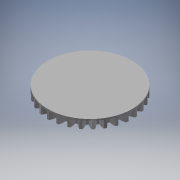
# Autodesk Inventor part: Stirnzahnrad1
Saved by Autodesk Inventor 2018 (Build 220112000, 112)
## iProperties
Created: 2018-01-27
Part Number: Stirnzahnrad1
Material: Steel
Document SubType Name: Modeling
Designer: gchri
Categories: <?xml version="1.0" encoding="UTF-16"?> <MemberInstance><Categories><FamilyTemplate><FamilyTemplateParameter ValueType="xs:double" Id="1" ObjectReferenceKey="da_z" ObjectType="kUserParameterObject"/><FamilyTemplateParameter ValueType="xs:double" Id="2" ObjectReferenceKey="da_b" ObjectType="kUserParameterObject"/><FamilyTemplateParameter ValueType="xs:double" Id="3" ObjectReferenceKey="da_beta" ObjectType="kUserParameterObject"/><FamilyTemplateParameter ValueType="xs:double" Id="4" ObjectReferenceKey="da_da" ObjectType="kUserParameterObject"/><FamilyTemplateParameter ValueType="xs:double" Id="5" ObjectReferenceKey="da_aw" ObjectType="kUserParameterObject"/><FamilyTemplateParameter ValueType="xs:string" Id="6" ObjectReferenceKey="EAIAABAAAACIAQAAAAAAAIAAAAAAAAAA" ObjectType="83910656" SubObjectId="SurfaceGeometry"/></FamilyTemplate><ParamToTemplateMap><ParamToTemplate CategoryParameter="//CategoryParameter[@InternalName='046C89C9-8512-4d59-83FE-43B91F4F132A']" TemplateParameter="1"/><ParamToTemplate CategoryParameter="//CategoryParameter[@InternalName='2552DF32-E462-4b46-AEBF-C6C7768E72AC']" TemplateParameter="2"/><ParamToTemplate CategoryParameter="//CategoryParameter[@InternalName='C9EE641D-15FC-4fae-A226-E94C4372FDD7']" TemplateParameter="3"/><ParamToTemplate><ParamToTemplate CategoryParameter="//CategoryParameter[@InternalName='00B6519A-459B-49c7-AD84-2E56D39A5744']" ConstantValue="0.000000"/></ParamToTemplate><ParamToTemplate><ParamToTemplate CategoryParameter="//CategoryParameter[@InternalName='04B31F0E-C7A6-4894-AA32-9629BEFACF47']" ConstantValue="1.000000"/></ParamToTemplate><ParamToTemplate><ParamToTemplate CategoryParameter="//CategoryParameter[@InternalName='43CBEC2E-7847-49e7-A936-2F7889FCB2D9']" ConstantValue="0.250000"/></ParamToTemplate><ParamToTemplate><ParamToTemplate CategoryParameter="//CategoryParameter[@InternalName='B1EFC894-105D-4ebd-86BF-FA20ED196853']" ConstantValue="0.350000"/></ParamToTemplate><ParamToTemplate><ParamToTemplate CategoryParameter="//CategoryParameter[@InternalName='51175063-3D10-4879-93E8-6246FE8B403D']" ConstantValue="2060000000.000000"/></ParamToTemplate><ParamToTemplate><ParamToTemplate CategoryParameter="//CategoryParameter[@InternalName='A3A52E27-4454-46a9-B0BD-C932399B70AF']" ConstantValue="0.300000"/></ParamToTemplate><ParamToTemplate><ParamToTemplate CategoryParameter="//CategoryParameter[@InternalName='91B76062-C214-41d9-B1B9-14D2AB99603D']" ConstantValue="0.175000"/></ParamToTemplate><ParamToTemplate><ParamToTemplate CategoryParameter="//CategoryParameter[@InternalName='374E806E-8B8A-4dda-A9AA-1039D6500AD2']" ConstantValue="5.714286"/></ParamToTemplate><ParamToTemplate><ParamToTemplate CategoryParameter="//CategoryParameter[@InternalName='2D373A89-B862-43d6-8D0B-0CBF12AB9F6C']" ConstantValue="0.349066"/></ParamToTemplate><ParamToTemplate CategoryParameter="//CategoryParameter[@InternalName='37777632-D6A2-4fac-9D53-DB8ACD95C989']" TemplateParameter="4"/><ParamToTemplate CategoryParameter="//CategoryParameter[@InternalName='FD1017F1-B727-4f7e-9707-0F86F1FF9423']" TemplateParameter="5"/><ParamToTemplate><ParamToTemplate CategoryParameter="//CategoryParameter[@InternalName='9E1B4470-B2D3-4ff1-B813-535BB4CDF51A']" ConstantValue="3520000.000000"/></ParamToTemplate><ParamToTemplate><ParamToTemplate CategoryParameter="//CategoryParameter[@InternalName='F8452263-BFF6-458c-9FB1-07C4B99E95CD']" ConstantValue="11400000.000000"/></ParamToTemplate><ParamToTemplate><ParamToTemplate CategoryParameter="//CategoryParameter[@InternalName='3E3BB259-FD49-497f-8171-6EBC954A3479']" ConstantValue="2.000000"/></ParamToTemplate><ParamToTemplate CategoryParameter="//CategoryParameter[@InternalName='27C3BAF2-7550-4e4b-AE2C-0DB134B7D9B7']" TemplateParameter="6"/></ParamToTemplateMap><Category DisplayName="Gear" InternalName="DC85795E-93AB-48d5-8EEE-5A27447B64BD" Mnemonic="Gear"><CategoryParameter DisplayName="z" InternalName="046C89C9-8512-4d59-83FE-43B91F4F132A" Mnemonic="z"/><CategoryParameter DisplayName="b" InternalName="2552DF32-E462-4b46-AEBF-C6C7768E72AC" Mnemonic="b"/><CategoryParameter DisplayName="||b|" InternalName="C9EE641D-15FC-4fae-A226-E94C4372FDD7" Mnemonic="beta"/><CategoryParameter DisplayName="x" InternalName="00B6519A-459B-49c7-AD84-2E56D39A5744" Mnemonic="x"/><CategoryParameter DisplayName="a*" InternalName="04B31F0E-C7A6-4894-AA32-9629BEFACF47" Mnemonic="a"/><CategoryParameter DisplayName="c*" InternalName="43CBEC2E-7847-49e7-A936-2F7889FCB2D9" Mnemonic="c"/><CategoryParameter DisplayName="r|.f|*" InternalName="B1EFC894-105D-4ebd-86BF-FA20ED196853" Mnemonic="rf"/><CategoryParameter DisplayName="E" InternalName="51175063-3D10-4879-93E8-6246FE8B403D" Mnemonic="E"/><CategoryParameter DisplayName="||m|" InternalName="A3A52E27-4454-46a9-B0BD-C932399B70AF" Mnemonic="mi"/><Category DisplayName="SpurGear" InternalName="26C5A22E-A91E-4dfd-A3B3-23CCAFAE1764" Mnemonic="SpurGear"><CategoryParameter DisplayName="m" InternalName="91B76062-C214-41d9-B1B9-14D2AB99603D" Mnemonic="m"/><CategoryParameter DisplayName="P" InternalName="374E806E-8B8A-4dda-A9AA-1039D6500AD2" Mnemonic="PP"/><CategoryParameter DisplayName="||a|" InternalName="2D373A89-B862-43d6-8D0B-0CBF12AB9F6C" Mnemonic="alpha"/><CategoryParameter DisplayName="d|.a|" InternalName="37777632-D6A2-4fac-9D53-DB8ACD95C989" Mnemonic="da"/><CategoryParameter DisplayName="a|.w|" InternalName="FD1017F1-B727-4f7e-9707-0F86F1FF9423" Mnemonic="aw"/><CategoryParameter DisplayName="||s||.Flim|" InternalName="9E1B4470-B2D3-4ff1-B813-535BB4CDF51A" Mnemonic="sFlim"/><CategoryParameter DisplayName="||s||.Hlim|" InternalName="F8452263-BFF6-458c-9FB1-07C4B99E95CD" Mnemonic="sHlim"/><CategoryParameter DisplayName="Typ" InternalName="3E3BB259-FD49-497f-8171-6EBC954A3479" Mnemonic="type"/><CategoryParameter DisplayName="PitchDiameter" InternalName="27C3BAF2-7550-4e4b-AE2C-0DB134B7D9B7" Mnemonic="IDS_PITCHDIAM"/></Category></Category></Categories></MemberInstance>
Density: 1 g/cm^3
Appearance: Steel
CustomPartVersion: 1
d16: 40,000 mm
d17: 0,000 mm
d41: 0,000 mm
d43: 40,000 mm
d46: 40,000 mm
d47: 0,000 mm
d48: 0,000 mm
Author: gchri
Autodesk Inventor part; units mm, degrees
note: some values were not read from the file. Chosen so that the rebuilt part matches the saved one: second side of "Extrusion6".
sketch "Sketch1" plane through (0, 0, 0) normal (0, 0, 1) x (1, 0, 0)
  circle A0 centre (0, 0) radius 27.9645
  dimension "d0" = 55.9289
  constraints: 1 centre point
  measures "d0" diameter of A0
extrude "Extrusion1" add sketch "Sketch1" along normal blind 6
ref_plane "Work Plane2" through (0, 0, 3) normal (0, 0, 1) x (1, 0, 0)
sketch "Sketch2" plane through (0, 0, 0) normal (0, 0, -1) x (-1, 0, 0)
  circle A0 centre (0, 0) radius 27.9645 projected
  circle A1 centre (0, 0) radius 26.6667
  dimension "d3" = 53.3333
  constraints: 1 centre point, 1 coincident
  measures "d3" diameter of A1
surface extrude "Flankendurchmesser" sketch "Sketch2" against normal through all shown no curves A1
ref_plane "Work Plane8" through (0, 0, 0) normal (0.9945219, 0.1045285, 0) x (0, 0, 1)
ref_plane "Work Plane9" through (0, 0, 0) normal (1, 0, 0) x (0, 1, 0)
spur gear teeth "Stirnzahnrad" teeth 30 pitch diameter 52.5 tip diameter 55.9289 root diameter 48.125 face width 5 start plane through (0, 0, 0) normal (0, 0, -1) x (-1, 0, 0)
sketch "Skizze9" plane through (0, 0, 6) normal (0, 0, 1) x (1, 0, 0)
  circle A0 centre (0, 40) radius 1.25 projected
  line L0 (5.4599, 22.7057) -> (-6.5384, 22.9075) projected
  line L1 (-6.5384, 22.9075) -> (-6.1348, 46.9042) projected
  line L2 (-6.1348, 46.9042) -> (5.8635, 46.7023) projected
  line L3 (5.8635, 46.7023) -> (5.4599, 22.7057) projected
  line L4 (-14.9485, 58.054) -> (-16.0417, -6.9368) projected
  line L5 (-16.0417, -6.9368) -> (13.9541, -7.4414) projected
  line L6 (15.0473, 57.5494) -> (13.9541, -7.4414) projected
  line L7 (-14.9485, 58.054) -> (15.0473, 57.5494) projected
  circle A1 centre (0, 0) radius 27.9645 projected
  line L8 (-29.0398, -6.7174) -> (27.9521, -7.6776)
  line L9 (27.9521, -7.6776) -> (28.4144, 12.3224)
  line L10 (-29.0398, -6.7174) -> (-28.5775, 13.2826)
  line L11 (-28.5775, 13.2826) -> (28.4144, 12.3224)
  dimension "d83" = 47.2
  dimension "d84" = 14
  dimension "d85" = 13
  dimension "d86" = 20
  dimension "d87" = 20
  constraints: 8 end point
  measures "d83" distance from line of A0.centre L8
  measures "d84" distance from line of L6 L8.end
  measures "d85" distance from line of L8.start L4
  measures "d86" vertical distance of L8.start L10.end
  measures "d87" vertical distance of L8.end L9.end
extrude "Extrusion6" add sketch "Skizze9" along normal blind 30 contours L11 A1 L8 L6 | L6 L5 L4 L11 | L11 L9 L8 A1 | L4 L8 A1 L11 | A1 L8 L10 L11
sketch "Skizze10" plane through (0, 0, 6) normal (0, 0, 1) x (1, 0, 0)
  line L0 (26.895, -7.6598) -> (-27.1377, -6.7495) projected
  arc A0 (-27.1377, -6.7495) -> (26.895, -7.6598) centre (0, 0) ccw projected
extrude "Extrusion7" cut sketch "Skizze10" against normal blind 30
sketch "Skizze11" plane through (0, 0, 36) normal (0, 0, 1) x (1, 0, 0)
  line L0 (-29.0398, -6.7174) -> (27.9521, -7.6776) projected
  line L1 (27.9521, -7.6776) -> (28.4144, 12.3224) projected
  line L2 (28.4144, 12.3224) -> (-28.5775, 13.2826) projected
  line L3 (-28.5775, 13.2826) -> (-29.0398, -6.7174) projected
  line L4 (5.4599, 22.7057) -> (-6.5384, 22.9075) projected
  line L5 (-6.5384, 22.9075) -> (-6.1348, 46.9042) projected
  line L6 (-6.1348, 46.9042) -> (5.8635, 46.7023) projected
  line L7 (5.8635, 46.7023) -> (5.4599, 22.7057) projected
  line L8 (-14.9485, 58.054) -> (-16.0417, -6.9368) projected
  line L9 (-16.0417, -6.9368) -> (13.9541, -7.4414) projected
  line L10 (15.0473, 57.5494) -> (13.9541, -7.4414) projected
  line L11 (-14.9485, 58.054) -> (15.0473, 57.5494) projected
  line L12 (28.4144, 12.3224) -> (-28.5775, 13.2826) projected
  line L13 (-6.1348, 12.9044) -> (14.2905, 12.5603)
  line L14 (-29.0398, -6.7174) -> (27.9521, -7.6776) projected
  line L15 (14.2905, 12.5603) -> (13.9541, -7.4414)
  line L16 (13.9541, -7.4414) -> (-16.0417, -6.9368)
  line L17 (-16.0417, -6.9368) -> (-15.7052, 13.0657)
  line L18 (-15.7052, 13.0657) -> (-6.1348, 12.9044)
  line L19 (-29.0398, -6.7174) -> (-28.5775, 13.2826) projected
  line L20 (-15.7052, 13.0657) -> (-28.5775, 13.2826)
  line L21 (-28.5775, 13.2826) -> (-28.5775, 13.2826)
  line L22 (-29.0398, -6.7174) -> (-16.0417, -6.9368)
  line L23 (14.2905, 12.5603) -> (28.4144, 12.3224)
  line L24 (28.4144, 12.3224) -> (27.9521, -7.6776) projected
  line L25 (27.9521, -7.6776) -> (13.9541, -7.4414)
  point P0 (0, 0)
  point P1 (14.2905, 12.5603)
  constraints: 20 end point, 7 point on line, 3 collinear
extrude "Extrusion8" cut sketch "Skizze11" against normal blind 30 contours L3 L2 L8 L0 | L10 L2 L1 L0
sketch "Skizze12" plane through (27.9521, -7.6776, 36) normal (0.0168745, 0.9998576, 0) x (0.9998576, -0.0168745, 0)
  line L0 (0, 0) -> (-14, 0) projected
  line L1 (0, 30) -> (0, 0) projected
  line L2 (-1.0573, 30) -> (0, 30) projected
  line L3 (-1.0573, 30) -> (-14, 30) projected
  line L4 (-14, 0) -> (-14, 30) projected
  point P0 (-28.0777, 36)
extrude "Extrusion9" cut sketch "Skizze12" against normal blind 30
sketch "Skizze13" plane through (0, 0, 36) normal (0, 0, 1) x (1, 0, 0)
  line L0 (13.9541, -7.4418) -> (13.9541, -7.4414) projected
  line L1 (13.9541, -7.4414) -> (14.2905, 12.5603) projected
  line L2 (14.2905, 12.5603) -> (-15.7052, 13.0657) projected
  line L3 (-15.7052, 13.0657) -> (-16.0417, -6.9364) projected
  line L4 (-16.0417, -6.9364) -> (13.9541, -7.4418) projected
  point P0 (0, 0)
extrude "Extrusion10" cut sketch "Skizze13" against normal blind 15
sketch "Skizze14" plane through (-25.3238, -6.78, 0) normal (-0.0168456, -0.9998581, 0) x (0.9998581, -0.0168456, 0)
  line L0 (39.2835, 21) -> (9.2835, 21) projected
  line L1 (9.2835, 21) -> (9.2835, 6) projected
  line L2 (9.2835, 6) -> (-1.8142, 6) projected
  line L3 (-1.8142, 5) -> (-1.8142, 6) projected
  line L4 (0, 5) -> (-1.8142, 5) projected
  line L5 (0, 0) -> (0, 5) projected
  line L6 (51.8032, 0) -> (0, 0) projected
  line L7 (51.8032, 5) -> (51.8032, 0) projected
  line L8 (52.2262, 5) -> (51.8032, 5) projected
  line L9 (52.2262, 6) -> (52.2262, 5) projected
  line L10 (52.2262, 6) -> (39.2835, 6) projected
  line L11 (39.2835, 6) -> (39.2835, 21) projected
  circle A0 centre (34.2835, 13.5) radius 1.7
  circle A1 centre (14.2835, 13.5) radius 1.7
  point P0 (25.206, 0)
  dimension "d100" = 3.4
  dimension "d101" = 3.4
  dimension "d102" = 5
  dimension "d103" = 5
  dimension "d104" = 7.5
  dimension "d105" = 7.5
  constraints: 2 centre point
  measures "d100" diameter of A0
  measures "d101" diameter of A1
  measures "d102" distance from line of L11 A0.centre
  measures "d103" distance from line of L1 A1.centre
  measures "d104" distance from line of L0 A1.centre
  measures "d105" distance from line of L0 A0.centre
extrude "Extrusion11" cut sketch "Skizze14" against normal blind 25 contours A0 | A1
sketch "Skizze15" plane through (0, 0, 21) normal (0, 0, 1) x (1, 0, 0)
  arc A0 (26.895, -7.6598) -> (-27.1377, -6.7495) centre (0, 0) ccw projected
  circle A1 centre (0, 0) radius 2.5
  dimension "d108" = 5
  constraints: 1 centre point, 1 coincident
  measures "d108" diameter of A1
extrude "Extrusion12" cut sketch "Skizze15" against normal through all
equation "\"d0\" = da_da"
equation "\"d3\" = da_dw"
equation "\"d16\" = da_aw"
equation "\"d43\" = da_aw"
equation "\"d46\" = da_aw"
equation "\"da_da\" = 55.928942"
equation "\"da_dw\" = 53.333333"
equation "\"da_aw\" = 40"
body "Solid1"
body "Srf1"
